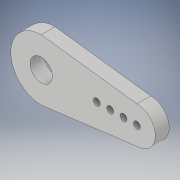
# Autodesk Inventor part: Servo horn
Saved by Autodesk Inventor 2019 (Build 230136000, 136)
## iProperties
Created: 2019-11-23
Part Number: Servo horn
Material: Generic
Document SubType Name: Modeling
Designer: User
Density: 1 g/cm^3
Appearance: Default
Author: User
Autodesk Inventor part; units mm, degrees
ref_plane "YZ Plane" through (0, 0, 0) normal (1, 0, 0) x (0, 1, 0)
ref_plane "XZ Plane" through (0, 0, 0) normal (0, 1, 0) x (-1, 0, 0)
ref_plane "XY Plane" through (0, 0, 0) normal (0, 0, 1) x (1, 0, 0)
sketch "Sketch1" plane through (0, 0, 0) normal (0, 0, 1) x (1, 0, 0)
  circle A0 centre (0, 0) radius 6.9469
  circle A1 centre (21.844, 0) radius 4.191
  line L0 (0, 6.9469) -> (21.844, 4.191)
  line L1 (0, -6.9469) -> (21.844, -4.191)
  dimension "d0" = 13.8938
  dimension "d1" = 8.382
  dimension "d2" = 21.844
  constraints: 4 end point, 4 point on circle, 2 centre point, 1 coincident
  measures "d0" diameter of A0
  measures "d1" diameter of A1
  measures "d2" distance of A1.centre point (0, 0)
extrude "Extrusion1" add sketch "Sketch1" along normal blind 3.175 contours L0 A0 L1 | L0 A1 L1 A0 | A1
sketch "Sketch2" plane through (0, 0, 3.175) normal (0, 0, 1) x (1, 0, 0)
  circle A0 centre (0, 0) radius 2.54
  circle A1 centre (12.7, 0) radius 0.7874
  circle A2 centre (15.748, 0) radius 0.7874
  circle A3 centre (18.796, 0) radius 0.7874
  circle A4 centre (21.844, 0) radius 0.7874
  dimension "d5" = 5.08
  dimension "d6" = 1.5748
  dimension "d7" = 1.5748
  dimension "d8" = 1.5748
  dimension "d9" = 1.5748
  dimension "d10" = 12.7
  dimension "d11" = 15.748
  dimension "d12" = 18.796
  dimension "d13" = 21.844
  constraints: 5 centre point, 1 coincident
  measures "d5" diameter of A0
  measures "d6" diameter of A1
  measures "d7" diameter of A2
  measures "d8" diameter of A3
  measures "d9" diameter of A4
  measures "d10" distance of A1.centre point (0, 0)
  measures "d11" distance of point (0, 0) A2.centre
  measures "d12" distance of point (0, 0) A3.centre
  measures "d13" distance of point (0, 0) A4.centre
extrude "Extrusion2" cut sketch "Sketch2" against normal blind 3.175
body "Solid1"
